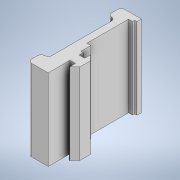
# Autodesk Inventor part: Tape_Belt_Layer
Saved by Autodesk Inventor 2021 (Build 250183000, 183)
## iProperties
Created: 2021-08-10
Part Number: Tape_Belt_Layer
Material: Generic
Document SubType Name: Modeling
Designer: Jorian Brusind
Density: 1 g/cm^3
Appearance: Default
Author: Jorian Brusind
Autodesk Inventor part; units mm, degrees
ref_plane "YZ Plane" through (0, 0, 0) normal (1, 0, 0) x (0, 1, 0)
ref_plane "XZ Plane" through (0, 0, 0) normal (0, 1, 0) x (-1, 0, 0)
ref_plane "XY Plane" through (0, 0, 0) normal (0, 0, 1) x (1, 0, 0)
sketch "Sketch1" plane through (0, 0, 0) normal (0, 1, 0) x (-1, 0, 0)
  line L0 (-5, -23) -> (5, -23)
  line L1 (5, -23) -> (5, 23)
  line L2 (5, 23) -> (-5, 23)
  line L3 (-5, 23) -> (-5, -23)
  line L4 (-5, -23) -> (5, 23) construction
  line L5 (5, -23) -> (-5, 23) construction
  point P0 (0, 0)
  dimension "d0" = 10
  dimension "d1" = 46
  constraints: 12 end point, 2 midpoint, 2 parallel, 1 horizontal, 1 perpendicular
  measures "d0" distance of L2.end L1.end
  measures "d1" distance of L1.end L0.end
extrude "Extrusion1" add sketch "Sketch1" along normal blind 40
sketch "Sketch2" plane through (0, 40, 0) normal (0, 1, 0) x (1, 0, 0)
  line L0 (5, -23) -> (5, 23) projected
  line L1 (5, 23) -> (-5, 23) projected
  line L2 (5, 23) -> (4.4285, 23)
  line L3 (4.4285, 23) -> (4.4285, 7.3)
  line L4 (3.857, 20.3) -> (5, 20.3)
  line L5 (5, 20.3) -> (5, -5.7)
  line L6 (5, -5.7) -> (3.857, -5.7)
  line L7 (3.857, -5.7) -> (3.857, 20.3)
  line L8 (3.857, 20.3) -> (5, -5.7) construction
  line L9 (5, 20.3) -> (3.857, -5.7) construction
  point P0 (5, -5.7)
  point P1 (5, 20.3)
  dimension "d7" = 0.5715
  dimension "d8" = 15.7
  dimension "d9" = 90
  dimension "d10" = 1.143
  dimension "d11" = 26
  constraints: 16 end point, 2 midpoint, 2 parallel, 2 perpendicular, 1 horizontal, 1 point on line
  measures "d7" distance of L0.end L2.end
  measures "d8" distance of L2.end L3.end
  measures "d9" angle of L3 L2
  measures "d10" distance of L5.end L6.end
  measures "d11" distance of L4.end L5.end
extrude "Extrusion2" cut sketch "Sketch2" against normal through all contours L6 L7 L4 L0
sketch "Sketch3" plane through (0, 40, 0) normal (0, 1, 0) x (1, 0, 0)
  line L0 (3.857, -5.7) -> (3.857, 20.3) projected
  line L1 (3.857, 9.5) -> (2.857, 9.5)
  line L2 (1.857, 19.75) -> (3.857, 19.75)
  line L3 (3.857, 19.75) -> (3.857, -0.75)
  line L4 (3.857, -0.75) -> (1.857, -0.75)
  line L5 (1.857, -0.75) -> (1.857, 19.75)
  line L6 (1.857, 19.75) -> (3.857, -0.75) construction
  line L7 (3.857, 19.75) -> (1.857, -0.75) construction
  line L8 (5, 23) -> (-5, 23) projected
  point P0 (3.857, -0.75)
  point P1 (3.857, 19.75)
  dimension "d51" = 1
  dimension "d53" = 2
  dimension "d54" = 20.5
  dimension "d59" = 2
  dimension "d60" = 90
  dimension "d61" = 13.5
  constraints: 14 end point, 2 midpoint, 2 parallel, 1 horizontal, 1 perpendicular
  measures "d51" distance of L1.start L1.end
  measures "d53" distance of L3.end L4.end
  measures "d54" distance of L2.end L3.end
  measures "d59" distance between parallel lines of L0 L5
  measures "d60" angle of L0 L1
  measures "d61" distance from line of L8 L1.end
sketch "Sketch4" plane through (0, 40, 0) normal (0, 1, 0) x (1, 0, 0)
  line L0 (5, -23) -> (5, -5.7) projected
  line L1 (5, -23) -> (5, -10)
  line L2 (5, -10) -> (7, -10)
  line L3 (7, -10) -> (7, -16)
  line L4 (7, -10) -> (7, -4)
  line L5 (7, -10) -> (11, -10)
  line L6 (11, -10) -> (11, -12.9395)
  line L7 (11, -10) -> (11, -7.06)
  line L8 (7, -16) -> (7.939, -16)
  line L9 (7, -4) -> (7.939, -4)
  line L10 (7.939, -4) -> (11, -7.06)
  line L11 (11, -12.9395) -> (7.939, -16)
  line L12 (7, -10) -> (7, -13)
  line L13 (7, -10) -> (7, -7)
  line L14 (7, -10) -> (10, -10) construction
  line L15 (7, -7) -> (5, -7)
  line L16 (7, -13) -> (5, -13)
  line L17 (5, -13) -> (5, -7)
  line L18 (7.75, -10.95) -> (7.75, -15.25)
  line L19 (7.75, -15.25) -> (7.6284, -15.25)
  line L20 (7.6284, -15.25) -> (10.25, -12.6288)
  line L21 (10.25, -12.6288) -> (10.25, -13)
  line L22 (10.25, -13) -> (10.25, -7.3707)
  line L23 (10.25, -7.3707) -> (7.6284, -4.75)
  line L24 (7.6284, -4.75) -> (7.75, -4.75)
  line L25 (7.75, -4.75) -> (7.75, -10.25)
  line L26 (7.75, -13.1) -> (9.95, -13.1) construction
  line L27 (7.75, -7.5) -> (9.65, -7.5) construction
  line L28 (5, -23) -> (5, -5.7) projected
  line L29 (7.75, -10.95) -> (7.75, -10.25)
  line L30 (6, -13) -> (6, -12.25)
  line L31 (6, -12.25) -> (7.75, -12.25)
  line L32 (6, -12.25) -> (5, -12.25)
  line L33 (6, -7) -> (6, -7.75)
  line L34 (6, -7.75) -> (5, -7.75)
  line L35 (6, -7.75) -> (7.75, -7.75)
  point P0 (0, 0)
  point P1 (5, -7)
  point P2 (7, -7.1)
  point P3 (7.75, -10)
  point P4 (10.25, -10)
  point P5 (10.25, -13)
  point P6 (5, -7.75)
  point P7 (7.75, -10.75)
  point P8 (7.75, -4.8715)
  point P9 (7.75, -15.1284)
  dimension "d19" = 13
  dimension "d20" = 2
  dimension "d21" = 6
  dimension "d22" = 6
  dimension "d23" = 4
  dimension "d24" = 2.9395
  dimension "d25" = 2.94
  dimension "d26" = 0.939
  dimension "d27" = 0.939
  dimension "d28" = 3
  dimension "d29" = 3
  dimension "d30" = 90
  dimension "d31" = 0.75
  dimension "d32" = 0.75
  dimension "d47" = 0.75
  dimension "d48" = 0.75
  constraints: 68 end point, 9 point on line, 7 horizontal, 7 perpendicular, 5 midpoint, 4 vertical, 2 collinear, 6 other
  measures "d19" distance of L0.start L1.end
  measures "d20" distance of L1.end L2.end
  measures "d21" distance of L2.end L3.end
  measures "d22" distance of L2.end L4.end
  measures "d23" distance of L2.end L5.end
  measures "d24" distance of L5.end L6.end
  measures "d25" distance of L5.end L7.end
  measures "d26" distance of L3.end L8.end
  measures "d27" distance of L4.end L9.end
  measures "d28" distance of L2.end L12.end
  measures "d29" distance of L2.end L13.end
  measures "d30" angle of L14 L13
  measures "d31" distance between parallel lines of L11 L20
  measures "d32" distance between parallel lines of L10 L23
  measures "d47" distance of L30.start L30.end
  measures "d48" distance of L33.start L33.end
extrude "Extrusion5" add sketch "Sketch4" against normal up to surface (40 mm away) contours L0 L2 L3 L31 L32 | L0 L34 L35 L4 L2 | L18 L19 L20 | L5 L25 L29 L18 L31 L3 | L4 L35 L25 L5 | L25 L23 L22 L5 | L5 L22 L20 L18 L29 L25
sketch "Sketch5" plane through (0, 40, 0) normal (0, 1, 0) x (1, 0, 0)
  line L0 (-8.5, 16.5) -> (-1.5, 16.5)
  line L1 (-1.5, 16.5) -> (-1.5, -16.5)
  line L2 (-1.5, -16.5) -> (-8.5, -16.5)
  line L3 (-8.5, -16.5) -> (-8.5, 16.5)
  line L4 (-5, 23) -> (-5, -23) projected
  line L5 (-8.5, 16.5) -> (-1.5, -16.5) construction
  line L6 (-1.5, 16.5) -> (-8.5, -16.5) construction
  point P0 (0, 0)
  point P1 (-5, 0)
  point P2 (-5, 16.5)
  point P3 (-5, -16.5)
  dimension "d41" = 7
  dimension "d42" = 33
  constraints: 12 end point, 3 midpoint, 2 parallel, 1 horizontal, 1 perpendicular
  measures "d41" distance of L1.end L2.end
  measures "d42" distance of L0.end L1.end
extrude "Extrusion6" cut sketch "Sketch5" against normal through all contours L0 L1 L2 L4
fillet "Fillet1" radius 1.75 4 edges at (-5, 20, 16.5) (-5, 20, 23) (-5, 20, -16.5) (-5, 20, -23)
fillet "Fillet2" radius 1.75 2 edges at (-1.5, 20, -16.5) (-1.5, 20, 16.5)
move faces "Move3" translate (0, 0, -0.5) faces at (4.619, 26.6667, -20.3)
extrude "Extrusion7" cut sketch "Sketch3" against normal through all
body "Solid1"
